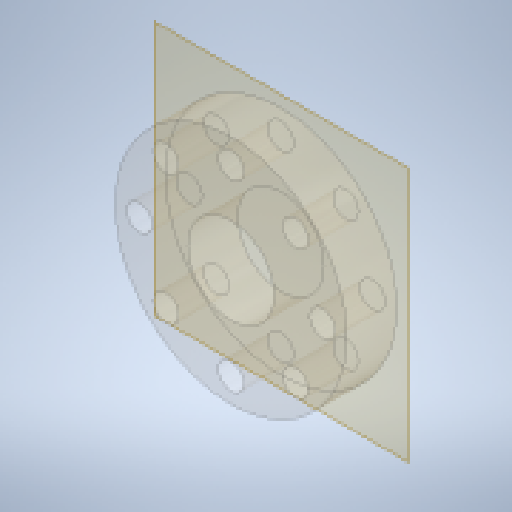
# Autodesk Inventor part: 64horn
Saved by Autodesk Inventor 2024 (Build 280153000, 153)
## iProperties
Created: 2024-09-07
Part Number: 64horn
Material: PMMA 플라스틱
Document SubType Name: Modeling
Designer: Eungang
Density: 1.188 g/cm^3
Appearance: 폴리카보네이트 - 선명
Author: Eungang
Autodesk Inventor part; units mm, degrees
ref_plane "YZ Plane" through (0, 0, 0) normal (1, 0, 0) x (0, 1, 0)
ref_plane "XZ Plane" through (0, 0, 0) normal (0, 1, 0) x (-1, 0, 0)
ref_plane "XY Plane" through (0, 0, 0) normal (0, 0, 1) x (1, 0, 0)
ref_plane "작업 평면1" through (0, 0, 0) normal (0, 0, 1) x (1, 0, 0)
sketch "스케치1" plane through (0, 0, 0) normal (0, 0, 1) x (1, 0, 0)
  circle A0 centre (-7.7782, -7.7782) radius 1.55 projected
  circle A1 centre (7.7782, -7.7782) radius 1.55 projected
  circle A2 centre (7.7782, 7.7782) radius 1.55 projected
  circle A3 centre (-7.7782, 7.7782) radius 1.55 projected
  circle A4 centre (0, 0) radius 5 projected
  circle A5 centre (0, 0) radius 13.9 projected
  circle A6 centre (0, 11) radius 1.55 projected
  circle A7 centre (11, 0) radius 1.55 projected
  circle A8 centre (0, -11) radius 1.55 projected
  circle A9 centre (-11, 0) radius 1.55 projected
  circle A10 centre (0, 0) radius 5.2
  circle A11 centre (0, 0) radius 13.9
  circle A12 centre (11, 0) radius 1.35
  circle A13 centre (7.7782, 7.7782) radius 1.35
  circle A14 centre (0, 11) radius 1.35
  circle A15 centre (-7.7782, 7.7782) radius 1.35
  circle A16 centre (-11, 0) radius 1.35
  circle A17 centre (-7.7782, -7.7782) radius 1.35
  circle A18 centre (0, -11) radius 1.35
  circle A19 centre (7.7782, -7.7782) radius 1.35
  dimension "d0" = 0.2
  dimension "d1" = 2.7
  dimension "d4" = 360
  constraints: 10 centre point, 2 coincident, 1 concentric, 17 other
  measures "d0" radial gap between concentric circles of A4 A10
  measures "d1" diameter of A12
extrude "돌출1" add sketch "스케치1" along normal blind 6 contours A5
